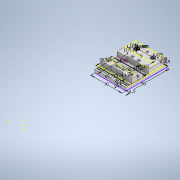
# Autodesk Inventor part: YAchseBasisteil
Saved by Autodesk Inventor 2021 (Build 250183000, 183)
## iProperties
Created: 2021-02-21
Part Number: YAchseBasisteil
Material: Generisch
Document SubType Name: Modeling
Designer: Kathrin H. Ulmer
Density: 1 g/cm^3
Appearance: Vorgabe
Author: Kathrin H. Ulmer
Autodesk Inventor part; units mm, degrees
ref_plane "YZ Plane" through (0, 0, 0) normal (1, 0, 0) x (0, 1, 0)
ref_plane "XZ Plane" through (0, 0, 0) normal (0, 1, 0) x (-1, 0, 0)
ref_plane "XY Plane" through (0, 0, 0) normal (0, 0, 1) x (1, 0, 0)
sketch "Skizze1" plane through (0, 0, 0) normal (0, 1, 0) x (-1, 0, 0)
  line L0 (28.961, -192.7131) -> (-41.039, -192.7131)
  line L1 (-41.039, -192.7131) -> (-41.039, -282.7131)
  line L2 (-41.039, -282.7131) -> (28.961, -282.7131)
  line L3 (28.961, -282.7131) -> (28.961, -192.7131)
  line L4 (28.961, -196.2131) -> (-41.039, -196.2131)
  line L5 (28.961, -204.2131) -> (-41.039, -204.2131)
  line L6 (28.961, -200.2131) -> (-41.039, -200.2131)
  line L7 (28.961, -246.7131) -> (-41.039, -246.7131)
  line L8 (28.961, -238.7131) -> (-41.039, -238.7131)
  line L9 (28.961, -242.7131) -> (-41.039, -242.7131)
  line L10 (28.961, -192.7131) -> (-41.039, -192.7131)
  line L11 (-41.039, -192.7131) -> (-41.039, -191.2131)
  line L12 (-41.039, -191.2131) -> (28.961, -191.2131)
  line L13 (28.961, -191.2131) -> (28.961, -192.7131)
  point P0 (0, 0)
  dimension "d0" = 70
  dimension "d1" = 90
  dimension "d206" = 3.5
  dimension "d207" = 8
  dimension "d220" = 4
  dimension "d221" = 54
  dimension "d222" = 8
  dimension "d223" = 4
  dimension "d255" = 36
  dimension "d282" = 70
  dimension "d283" = 1.5
  constraints: 28 end point, 12 point on line, 7 perpendicular, 4 parallel, 3 horizontal
  measures "d0" distance of L2.end L1.end
  measures "d1" distance of L1.end L0.end
  measures "d206" distance between parallel lines of L4 L0
  measures "d207" distance between parallel lines of L5 L4
  measures "d220" distance between parallel lines of L5 L6
  measures "d221" distance between parallel lines of L0 L7
  measures "d222" distance between parallel lines of L7 L8
  measures "d223" distance between parallel lines of L7 L9
  measures "d255" distance between parallel lines of L2 L7
  measures "d282" distance of L11.end L12.end
  measures "d283" distance of L10.end L11.end
extrude "Extrusion1" add sketch "Skizze1" along normal blind 7 contours L3 L4 L1 L0 | L3 L6 L1 L4 | L3 L5 L1 L6 | L3 L8 L1 L5 | L3 L9 L1 L8 | L3 L7 L1 L9 | L3 L2 L1 L7
sketch "Skizze2" plane through (0, 7, 0) normal (0, 1, 0) x (1, 0, 0)
  line L0 (41.039, 282.7131) -> (-28.961, 282.7131) projected
  line L1 (-28.961, 282.7131) -> (41.039, 282.7131)
  line L2 (41.039, 282.7131) -> (41.039, 258.7131)
  line L3 (41.039, 258.7131) -> (-28.961, 258.7131)
  line L4 (-28.961, 258.7131) -> (-28.961, 282.7131)
  circle A0 centre (-13.961, 268.7131) radius 4.5
  circle A1 centre (26.039, 268.7131) radius 4.5
  point P0 (0, 0)
  point P1 (41.039, 282.7131)
  dimension "d4" = 24
  dimension "d5" = 70
  dimension "d17" = 9
  dimension "d18" = 9
  dimension "d19" = 15
  dimension "d21" = 10
  dimension "d22" = 15
  dimension "d23" = 40
  dimension "d64" = 10
  constraints: 8 end point, 2 centre point, 2 parallel, 1 horizontal, 1 perpendicular
  measures "d4" distance of L1.end L2.end
  measures "d5" distance of L2.end L3.end
  measures "d17" diameter of A0
  measures "d18" diameter of A1
  measures "d19" distance from line of L4 A0.centre
  measures "d21" distance from line of L3 A1.centre
  measures "d22" distance from line of L2 A1.centre
  measures "d23" distance of A1.centre A0.centre
  measures "d64" distance from line of L3 A0.centre
extrude "Extrusion2" add sketch "Skizze2" along normal blind 10 contours L2 L3 L4 L0 | A0 | A1
sketch "Skizze4" plane through (0, 17, 0) normal (0, 1, 0) x (1, 0, 0)
  point P0 (0, 0)
sketch "Skizze5" plane through (-28.961, 7, -258.7131) normal (0, 0, 1) x (1, 0, 0)
  point P0 (28.961, -7)
sketch "Skizze6" plane through (0, 17, 0) normal (0, 1, 0) x (1, 0, 0)
  circle A0 centre (-11.961, 268.7131) radius 4.5
  line L0 (41.039, 282.7131) -> (-28.961, 282.7131) projected
  line L1 (-28.961, 282.7131) -> (-28.961, 258.7131) projected
  line L2 (-28.961, 258.7131) -> (41.039, 258.7131) projected
  point P0 (0, 0)
  dimension "d34" = 9
  dimension "d36" = 17
  dimension "d65" = 10
  constraints: 1 centre point
  measures "d34" diameter of A0
  measures "d36" distance from line of L1 A0.centre
  measures "d65" distance from line of L2 A0.centre
sketch "Skizze9" plane through (0, 17, 0) normal (0, 1, 0) x (1, 0, 0)
  point P0 (0, 0)
sketch "Skizze10" plane through (0, 17, 0) normal (0, 1, 0) x (1, 0, 0)
  circle A0 centre (24.039, 268.7131) radius 4.5
  line L0 (41.039, 258.7131) -> (41.039, 282.7131) projected
  line L1 (41.039, 282.7131) -> (-28.961, 282.7131) projected
  line L2 (-28.961, 282.7131) -> (-28.961, 258.7131) projected
  point P0 (0, 0)
  dimension "d37" = 9
  dimension "d38" = 17
  dimension "d39" = 14
  dimension "d40" = 70
  constraints: 1 centre point
  measures "d37" diameter of A0
  measures "d38" distance from line of L0 A0.centre
  measures "d39" distance from line of L1 A0.centre
  measures "d40" distance between parallel lines of L0 L2
sketch "Skizze11" plane through (0, 17, 0) normal (0, 1, 0) x (1, 0, 0)
  point P0 (0, 0)
extrude "Extrusion6" cut sketch "Skizze6" against normal blind 14
sketch "Skizze16" plane through (0, 17, 0) normal (0, 1, 0) x (1, 0, 0)
  line L0 (41.039, 282.7131) -> (-28.961, 282.7131) projected
  line L1 (-28.961, 258.7131) -> (41.039, 258.7131) projected
  point P0 (0, 0)
  dimension "d63" = 24
  measures "d63" distance between parallel lines of L0 L1
extrude "Extrusion11" cut sketch "Skizze10" against normal blind 13.75
sketch "Skizze17" plane through (41.039, 0, -192.7131) normal (1, 0, 0) x (0, 0, -1)
  line L0 (86.5, 13) -> (84, 13)
  line L1 (84, 13) -> (84, 7.5)
  line L2 (84, 7.5) -> (86.5, 7.5)
  line L3 (86.5, 7.5) -> (86.5, 13)
  line L4 (90, 0) -> (90, 17) projected
  line L5 (66, 17) -> (90, 17) projected
  point P0 (-192.7131, 0)
  dimension "d68" = 2.5
  dimension "d69" = 5.5
  dimension "d70" = 3.5
  dimension "d71" = 4
  constraints: 8 end point, 2 parallel, 1 horizontal, 1 perpendicular
  measures "d68" distance of L2.end L1.end
  measures "d69" distance of L1.end L0.end
  measures "d70" distance between parallel lines of L4 L3
  measures "d71" distance between parallel lines of L5 L0
extrude "Extrusion12" cut sketch "Skizze17" against normal blind 23
sketch "Skizze18" plane through (-28.961, 0, -282.7131) normal (-1, 0, 0) x (0, 0, 1)
  line L0 (3.5, 7.5) -> (6, 7.5)
  line L1 (6, 7.5) -> (6, 13)
  line L2 (6, 13) -> (3.5, 13)
  line L3 (3.5, 13) -> (3.5, 7.5)
  line L4 (0, 17) -> (24, 17) projected
  line L5 (0, 0) -> (0, 17) projected
  point P0 (282.7131, 0)
  dimension "d74" = 2.5
  dimension "d75" = 5.5
  dimension "d76" = 4
  dimension "d77" = 3.5
  constraints: 8 end point, 2 parallel, 1 horizontal, 1 perpendicular
  measures "d74" distance of L2.end L1.end
  measures "d75" distance of L1.end L0.end
  measures "d76" distance between parallel lines of L4 L2
  measures "d77" distance between parallel lines of L5 L3
extrude "Extrusion13" cut sketch "Skizze18" against normal blind 23
sketch "Skizze19" plane through (41.039, 0, -282.7131) normal (0, 0, -1) x (-1, 0, 0)
  circle A0 centre (53, 10.125) radius 2.125
  line L0 (70, 0) -> (70, 17) projected
  line L1 (0, 17) -> (70, 17) projected
  circle A1 centre (17, 10.125) radius 2.125
  line L2 (0, 0) -> (0, 17) projected
  point P0 (41.039, 0)
  dimension "d80" = 4.25
  dimension "d81" = 17
  dimension "d82" = 6.875
  dimension "d83" = 4.25
  dimension "d84" = 6.875
  dimension "d85" = 17
  constraints: 2 centre point
  measures "d80" diameter of A0
  measures "d81" distance from line of L0 A0.centre
  measures "d82" distance from line of L1 A0.centre
  measures "d83" diameter of A1
  measures "d84" distance from line of L1 A1.centre
  measures "d85" distance from line of L2 A1.centre
extrude "Extrusion14" cut sketch "Skizze19" against normal blind 30 contours A1
extrude "Extrusion15" cut sketch "Skizze19" against normal blind 30 contours A0
sketch "Skizze20" plane through (41.039, 0, -282.7131) normal (0, 0, -1) x (-1, 0, 0)
  circle A0 centre (8, 10.125) radius 2.25
  line L0 (0, 17) -> (70, 17) projected
  line L1 (0, 0) -> (0, 17) projected
  circle A1 centre (62, 10.125) radius 2.125
  line L2 (70, 0) -> (70, 17) projected
  point P0 (41.039, 0)
  dimension "d90" = 4.5
  dimension "d91" = 6.875
  dimension "d92" = 8
  dimension "d93" = 4.25
  dimension "d94" = 6.875
  dimension "d95" = 8
  constraints: 2 centre point
  measures "d90" diameter of A0
  measures "d91" distance from line of L0 A0.centre
  measures "d92" distance from line of L1 A0.centre
  measures "d93" diameter of A1
  measures "d94" distance from line of L0 A1.centre
  measures "d95" distance from line of L2 A1.centre
extrude "Extrusion16" cut sketch "Skizze20" against normal blind 30 contours A0
extrude "Extrusion17" cut sketch "Skizze20" against normal blind 30 contours A1
sketch "Skizze21" plane through (0, 7, 0) normal (0, 1, 0) x (1, 0, 0)
  line L0 (-28.961, 282.7131) -> (-28.961, 192.7131) projected
  line L1 (41.039, 192.7131) -> (41.039, 282.7131) projected
  line L2 (-86.883, 193.3511) -> (41.039, 193.3511)
  line L3 (41.039, 193.3511) -> (41.039, 216.8511)
  line L4 (41.039, 216.8511) -> (-86.883, 216.8511)
  line L5 (-86.883, 216.8511) -> (-86.883, 193.3511)
  line L6 (-86.883, 216.8511) -> (-16.883, 216.8511)
  line L7 (-16.883, 216.8511) -> (-16.883, 208.3511)
  line L8 (41.039, 206.8012) -> (-28.961, 206.8012)
  line L9 (-86.883, 208.3511) -> (-86.883, 216.8511)
  line L10 (-28.961, 206.8012) -> (-6.961, 206.8012)
  line L11 (-6.961, 206.8012) -> (-6.961, 204.8012)
  line L12 (-6.961, 204.8012) -> (-28.961, 204.8012)
  line L13 (-28.961, 204.8012) -> (-28.961, 206.8012)
  line L14 (41.039, 206.8012) -> (19.039, 206.8012)
  line L15 (19.039, 206.8012) -> (19.039, 204.8012)
  line L16 (19.039, 204.8012) -> (41.039, 204.8012)
  line L17 (41.039, 204.8012) -> (41.039, 206.8012)
  line L18 (-86.883, 204.8511) -> (41.039, 204.8511)
  line L19 (-86.883, 196.8511) -> (41.039, 196.8511)
  point P0 (0, 0)
  point P1 (41.039, 206.8012)
  point P2 (-28.961, 216.8511)
  point P3 (-28.961, 206.8012)
  point P4 (-28.961, 204.8012)
  point P5 (41.039, 204.8012)
  point P6 (41.039, 216.8511)
  dimension "d101" = 8.5
  dimension "d102" = 22
  dimension "d103" = 2
  dimension "d104" = 22
  dimension "d105" = 2
  dimension "d203" = 0.0499
  dimension "d204" = 8
  dimension "d205" = 3.5
  dimension "d286" = 13.4501
  constraints: 36 end point, 8 parallel, 6 perpendicular, 4 horizontal, 4 point on line
  measures "d101" distance of L7.end L6.end
  measures "d102" distance of L11.end L12.end
  measures "d103" distance between parallel lines of L12 L8
  measures "d104" distance of L16.end L15.end
  measures "d105" distance of L15.end L14.end
  measures "d203" distance between parallel lines of L12 L18
  measures "d204" distance between parallel lines of L18 L19
  measures "d205" distance between parallel lines of L2 L19
  measures "d286" distance between parallel lines of L2 L8
sketch "Skizze22" plane through (0, 7, 0) normal (0, 1, 0) x (1, 0, 0)
  line L0 (-22.961, 228.2131) -> (-17.861, 228.2131)
  line L1 (-17.861, 228.2131) -> (-17.861, 222.7131)
  line L2 (-17.861, 222.7131) -> (-22.961, 222.7131)
  line L3 (-22.961, 222.7131) -> (-22.961, 228.2131)
  line L4 (-3.861, 228.2131) -> (1.239, 228.2131)
  line L5 (1.239, 228.2131) -> (1.239, 222.7131)
  line L6 (1.239, 222.7131) -> (-3.861, 222.7131)
  line L7 (-3.861, 222.7131) -> (-3.861, 228.2131)
  line L8 (10.839, 228.2131) -> (15.939, 228.2131)
  line L9 (15.939, 228.2131) -> (15.939, 222.7131)
  line L10 (15.939, 222.7131) -> (10.839, 222.7131)
  line L11 (10.839, 222.7131) -> (10.839, 228.2131)
  line L12 (29.939, 228.2131) -> (35.039, 228.2131)
  line L13 (35.039, 228.2131) -> (35.039, 222.7131)
  line L14 (35.039, 222.7131) -> (29.939, 222.7131)
  line L15 (29.939, 222.7131) -> (29.939, 228.2131)
  line L16 (-28.961, 258.7131) -> (-28.961, 192.7131) projected
  line L17 (41.039, 192.7131) -> (41.039, 258.7131) projected
  line L18 (-28.961, 192.7131) -> (41.039, 192.7131) projected
  point P0 (0, 0)
  dimension "d120" = 5.1
  dimension "d121" = 5.5
  dimension "d122" = 5.1
  dimension "d123" = 5.1
  dimension "d124" = 5.1
  dimension "d125" = 6
  dimension "d126" = 6
  dimension "d127" = 14
  dimension "d128" = 14
  dimension "d161" = 30
  constraints: 32 end point, 8 parallel, 6 point on line, 4 horizontal, 4 perpendicular
  measures "d120" distance of L1.end L2.end
  measures "d121" distance of L0.end L1.end
  measures "d122" distance of L5.end L6.end
  measures "d123" distance of L9.end L10.end
  measures "d124" distance of L13.end L14.end
  measures "d125" distance between parallel lines of L16 L3
  measures "d126" distance between parallel lines of L17 L13
  measures "d127" distance between parallel lines of L15 L9
  measures "d128" distance between parallel lines of L1 L7
  measures "d161" distance between parallel lines of L18 L2
extrude "Extrusion22" add sketch "Skizze21" along normal blind 10 contours L4 L1 L8 L0
extrude "Extrusion23" add sketch "Skizze21" along normal blind 10 contours L8 L11 L18 L0 | L18 L11 L12 L0 | L8 L1 L18 L15 | L18 L1 L16 L15
sketch "Skizze25" plane through (0, 17, 0) normal (0, 1, 0) x (1, 0, 0)
  line L0 (-22.961, 214.8511) -> (-17.861, 214.8511)
  line L1 (-17.861, 214.8511) -> (-17.861, 210.6011)
  line L2 (-17.861, 210.6011) -> (-22.961, 210.6011)
  line L3 (-22.961, 210.6011) -> (-22.961, 214.8511)
  line L4 (-3.861, 214.8511) -> (1.239, 214.8511)
  line L5 (1.239, 214.8511) -> (1.239, 210.6011)
  line L6 (1.239, 210.6011) -> (-3.861, 210.6011)
  line L7 (-3.861, 210.6011) -> (-3.861, 214.8511)
  line L8 (10.839, 214.8511) -> (15.939, 214.8511)
  line L9 (15.939, 214.8511) -> (15.939, 210.6011)
  line L10 (15.939, 210.6011) -> (10.839, 210.6011)
  line L11 (10.839, 210.6011) -> (10.839, 214.8511)
  line L12 (29.939, 214.8511) -> (35.039, 214.8511)
  line L13 (35.039, 214.8511) -> (35.039, 210.6011)
  line L14 (35.039, 210.6011) -> (29.939, 210.6011)
  line L15 (29.939, 210.6011) -> (29.939, 214.8511)
  line L16 (-28.961, 216.8511) -> (-28.961, 204.8012) projected
  line L17 (41.039, 204.8012) -> (41.039, 216.8511) projected
  line L18 (41.039, 216.8511) -> (-28.961, 216.8511) projected
  point P0 (0, 0)
  point P1 (41.039, 216.2131)
  dimension "d141" = 5.1
  dimension "d142" = 4.25
  dimension "d143" = 5.1
  dimension "d144" = 4.25
  dimension "d145" = 5.1
  dimension "d146" = 4.25
  dimension "d147" = 5.1
  dimension "d148" = 4.25
  dimension "d149" = 6
  dimension "d150" = 14
  dimension "d151" = 6
  dimension "d152" = 14
  dimension "d153" = 2
  dimension "d154" = 2
  dimension "d155" = 2
  constraints: 32 end point, 8 parallel, 4 horizontal, 4 perpendicular, 1 point on line, 1 other
  measures "d141" distance of L1.end L2.end
  measures "d142" distance of L0.end L1.end
  measures "d143" distance of L5.end L6.end
  measures "d144" distance of L4.end L5.end
  measures "d145" distance of L9.end L10.end
  measures "d146" distance of L8.end L9.end
  measures "d147" distance of L13.end L14.end
  measures "d148" distance of L12.end L13.end
  measures "d149" distance between parallel lines of L16 L3
  measures "d150" distance between parallel lines of L7 L1
  measures "d151" distance between parallel lines of L17 L13
  measures "d152" distance between parallel lines of L9 L15
extrude "Extrusion24" cut sketch "Skizze25" against normal blind 30
sketch "Skizze27" plane through (0, 7, 0) normal (0, 1, 0) x (1, 0, 0)
  point P0 (0, 0)
sketch "Skizze28" plane through (0, 7, 0) normal (0, 1, 0) x (1, 0, 0)
  line L0 (-28.961, 258.7131) -> (-28.961, 216.8511) projected
  line L1 (41.039, 216.8511) -> (41.039, 258.7131) projected
  line L2 (-28.961, 253.3551) -> (41.039, 253.3551)
  line L3 (41.039, 253.3551) -> (41.039, 229.6051)
  line L4 (41.039, 229.6051) -> (-28.961, 229.6051)
  line L5 (-28.961, 229.6051) -> (-28.961, 253.3551)
  line L6 (41.039, 216.8511) -> (-28.961, 216.8511) projected
  line L7 (-28.961, 192.7131) -> (41.039, 192.7131) projected
  line L8 (-28.961, 204.8012) -> (-6.961, 204.8012) projected
  line L9 (-6.961, 206.8012) -> (19.039, 206.8012) projected
  line L10 (19.039, 204.8012) -> (41.039, 204.8012) projected
  line L11 (-28.961, 253.3551) -> (41.039, 253.3551)
  line L12 (41.039, 253.3551) -> (41.039, 244.8551)
  line L13 (41.039, 244.8551) -> (-28.961, 244.8551)
  line L14 (-28.961, 244.8551) -> (-28.961, 253.3551)
  line L15 (41.039, 204.8012) -> (41.039, 216.8511) projected
  line L16 (41.039, 244.8551) -> (19.039, 244.8551)
  line L17 (19.039, 244.8551) -> (19.039, 242.8551)
  line L18 (19.039, 242.8551) -> (41.039, 242.8551)
  line L19 (41.039, 242.8551) -> (41.039, 244.8551)
  line L20 (-28.961, 244.8551) -> (-6.961, 244.8551)
  line L21 (-6.961, 244.8551) -> (-6.961, 242.8551)
  line L22 (-6.961, 242.8551) -> (-28.961, 242.8551)
  line L23 (-28.961, 242.8551) -> (-28.961, 244.8551)
  point P0 (0, 0)
  point P1 (41.039, 253.3551)
  point P2 (-28.961, 242.8551)
  point P3 (41.039, 242.8551)
  point P4 (-28.961, 253.3551)
  dimension "d162" = 23.75
  dimension "d163" = 12.754
  dimension "d164" = 12.0881
  dimension "d165" = 14.0881
  dimension "d166" = 12.0499
  dimension "d167" = 8.5
  dimension "d168" = 10.0499
  dimension "d169" = 22
  dimension "d170" = 22
  dimension "d171" = 2
  dimension "d172" = 22
  dimension "d173" = 2
  dimension "d202" = 15.25
  constraints: 32 end point, 8 parallel, 4 horizontal, 4 perpendicular, 1 point on line
  measures "d162" distance between parallel lines of L4 L2
  measures "d163" distance between parallel lines of L4 L6
  measures "d164" distance between parallel lines of L7 L8
  measures "d165" distance between parallel lines of L7 L9
  measures "d166" distance between parallel lines of L10 L6
  measures "d167" distance between parallel lines of L13 L2
  measures "d168" distance between parallel lines of L9 L6
  measures "d169" distance from line of L10.start L15
  measures "d170" distance of L18.end L17.end
  measures "d171" distance of L17.end L16.end
  measures "d172" distance of L21.end L22.end
  measures "d173" distance of L20.end L21.end
  measures "d202" distance between parallel lines of L4 L13
sketch "Skizze30" plane through (0, 7, 0) normal (0, 1, 0) x (1, 0, 0)
  point P0 (0, 0)
extrude "Extrusion26" add sketch "Skizze28" along normal blind 10 contours L2 L1 L13 L0 | L13 L21 L22 L0 | L1 L18 L17 L13
sketch "Skizze31" plane through (0, 17, 0) normal (0, 1, 0) x (1, 0, 0)
  line L0 (-3.861, 33.1581) -> (1.239, 33.1581)
  line L1 (1.239, 33.1581) -> (1.239, 28.9081)
  line L2 (1.239, 28.9081) -> (-3.861, 28.9081)
  line L3 (-3.861, 28.9081) -> (-3.861, 33.1581)
  line L4 (10.839, 33.1581) -> (15.939, 33.1581)
  line L5 (15.939, 33.1581) -> (15.939, 28.9081)
  line L6 (15.939, 28.9081) -> (10.839, 28.9081)
  line L7 (10.839, 28.9081) -> (10.839, 33.1581)
  line L8 (41.039, 242.8551) -> (41.039, 253.3551) projected
  line L9 (-28.961, 253.3551) -> (-28.961, 242.8551) projected
  line L10 (-6.961, 204.8012) -> (-6.961, 206.8012) projected
  line L11 (19.039, 206.8012) -> (19.039, 204.8012) projected
  line L12 (19.039, 244.8551) -> (19.039, 242.8551) projected
  line L13 (-6.961, 242.8551) -> (-6.961, 244.8551) projected
  point P0 (0, 0)
  point P1 (-28.961, 250.7131)
  dimension "d190" = 5.1
  dimension "d191" = 4.25
  dimension "d192" = 5.1
  dimension "d193" = 4.25
  dimension "d194" = 25.1
  dimension "d195" = 25.1
  dimension "d196" = 26
  dimension "d197" = 26
  constraints: 16 end point, 4 parallel, 2 horizontal, 2 perpendicular
  measures "d190" distance of L1.end L2.end
  measures "d191" distance of L0.end L1.end
  measures "d192" distance of L5.end L6.end
  measures "d193" distance of L4.end L5.end
  measures "d194" distance between parallel lines of L8 L5
  measures "d195" distance between parallel lines of L9 L3
  measures "d196" distance between parallel lines of L10 L11
  measures "d197" distance between parallel lines of L12 L13
extrude "Extrusion28" cut sketch "Skizze31" against normal blind 30
extrude "Extrusion29" cut sketch "Skizze22" against normal blind 30
sketch "Skizze32" plane through (0, 17, 0) normal (0, 1, 0) x (1, 0, 0)
  line L0 (-3.861, 248.054) -> (1.239, 248.054)
  line L1 (1.239, 248.054) -> (1.239, 252.054)
  line L2 (1.239, 252.054) -> (-3.861, 252.054)
  line L3 (-3.861, 252.054) -> (-3.861, 248.054)
  line L4 (10.839, 248.054) -> (15.939, 248.054)
  line L5 (15.939, 248.054) -> (15.939, 252.054)
  line L6 (15.939, 252.054) -> (10.839, 252.054)
  line L7 (10.839, 252.054) -> (10.839, 248.054)
  line L8 (-28.961, 282.7131) -> (-28.961, 258.7131) projected
  line L9 (41.039, 258.7131) -> (41.039, 282.7131) projected
  line L10 (-6.961, 244.8551) -> (19.039, 244.8551) projected
  line L11 (-28.961, 242.4631) -> (41.039, 242.4631)
  line L12 (-28.961, 258.7131) -> (-28.961, 216.8511) projected
  line L13 (-6.961, 244.4631) -> (-6.961, 242.4631)
  line L14 (19.039, 244.4631) -> (19.039, 242.4631)
  line L15 (-10.545, 205.4869) -> (-10.545, 192.7131)
  line L16 (-28.961, 192.7131) -> (41.039, 192.7131) projected
  line L17 (-28.961, 199.3012) -> (41.039, 199.3012)
  line L18 (19.039, 204.8012) -> (41.039, 204.8012) projected
  line L19 (-28.961, 236.9631) -> (41.039, 236.9631)
  line L20 (-28.961, 258.7131) -> (41.039, 258.7131) projected
  line L21 (-6.961, 244.4631) -> (19.039, 244.4631)
  line L22 (-28.961, 258.7131) -> (41.039, 258.7131)
  line L23 (41.039, 258.7131) -> (41.039, 242.4631)
  line L24 (41.039, 242.4631) -> (-28.961, 242.4631)
  line L25 (-28.961, 242.4631) -> (-28.961, 258.7131)
  line L26 (-6.961, 244.4631) -> (19.039, 244.4631)
  line L27 (19.039, 244.4631) -> (19.039, 242.4631)
  line L28 (19.039, 242.4631) -> (-6.961, 242.4631)
  line L29 (-6.961, 242.4631) -> (-6.961, 244.4631)
  point P0 (0, 0)
  point P1 (-28.961, 242.8551)
  point P2 (41.039, 242.8551)
  dimension "d208" = 5.1
  dimension "d209" = 4
  dimension "d210" = 5.1
  dimension "d211" = 4
  dimension "d212" = 25.1
  dimension "d213" = 25.1
  dimension "d214" = 3.1988
  dimension "d215" = 3.1988
  dimension "d256" = 12.7738
  dimension "d257" = 5.5
  dimension "d258" = 5.5
  dimension "d259" = 37.6619
  dimension "d260" = 16.25
  dimension "d261" = 2
  constraints: 46 end point, 10 parallel, 7 horizontal, 4 perpendicular, 4 point on line
  measures "d208" distance of L2.end L1.end
  measures "d209" distance of L1.end L0.end
  measures "d210" distance of L6.end L5.end
  measures "d211" distance of L5.end L4.end
  measures "d212" distance between parallel lines of L8 L3
  measures "d213" distance between parallel lines of L9 L5
  measures "d214" distance between parallel lines of L10 L4
  measures "d215" distance from line of L0.end L10
  measures "d256" distance of L15.start L15.end
  measures "d257" distance between parallel lines of L18 L17
  measures "d258" distance between parallel lines of L19 L11
  measures "d259" distance between parallel lines of L17 L19
  measures "d260" distance between parallel lines of L20 L11
  measures "d261" distance between parallel lines of L11 L21
extrude "Extrusion30" cut sketch "Skizze32" against normal blind 30 contours L3 L2 L1 L0 | L7 L6 L5 L4
sketch "Skizze33" plane through (0, 17, 0) normal (0, 1, 0) x (1, 0, 0)
  line L0 (41.039, 216.8511) -> (-28.961, 216.8511) projected
  line L1 (-28.961, 192.7131) -> (41.039, 192.7131) projected
  line L2 (19.039, 242.8551) -> (41.039, 242.8551) projected
  point P0 (0, 0)
  point P1 (41.039, 216.2131)
  point P2 (-28.961, 216.8511)
  dimension "d218" = 24.138
  dimension "d219" = 50.142
  constraints: 1 other
  measures "d219" distance between parallel lines of L2 L1
sketch "Skizze34" plane through (0, 17, 0) normal (0, 1, 0) x (1, 0, 0)
  point P0 (0, 0)
sketch "Skizze35" plane through (41.039, 0, -282.7131) normal (0, 0, -1) x (-1, 0, 0)
  circle A0 centre (62, 10.125) radius 2.125 projected
  line L0 (62, 10.125) -> (62, 17)
  line L1 (0, 17) -> (70, 17) projected
  line L2 (53.0937, 10.125) -> (53.0937, 17)
  line L3 (17.1042, 10.125) -> (17.1042, 17)
  line L4 (62, 10.125) -> (70, 10.125)
  line L5 (53.0937, 10.125) -> (70, 10.125)
  line L6 (8.0195, 10.125) -> (0, 10.125)
  point P0 (41.039, 0)
  dimension "d141" = 5.1
  dimension "d142" = 4.25
  dimension "d143" = 5.1
  dimension "d144" = 4.25
  dimension "d145" = 5.1
  dimension "d146" = 4.25
  dimension "d147" = 5.1
  dimension "d148" = 4.25
  dimension "d149" = 6
  dimension "d150" = 14
  dimension "d151" = 6
  dimension "d152" = 14
  dimension "d153" = 2
  dimension "d154" = 2
  dimension "d155" = 2
  dimension "d224" = 8
  dimension "d225" = 16.9063
  dimension "d226" = 8.0195
  dimension "d227" = 17.1042
  dimension "d229" = 6.875
  dimension "d230" = 6.875
  constraints: 12 end point, 3 point on line, 2 horizontal, 2 parallel, 1 vertical
  measures "d224" distance of L0.start L4.end
  measures "d225" distance of L2.start L4.end
  measures "d226" distance of L6.start L6.end
  measures "d227" distance of L6.end L3.start
  measures "d229" distance of L3.start L3.end
  measures "d230" distance of L2.start L2.end
sketch "Skizze36" plane through (-28.961, 0, -282.7131) normal (-1, 0, 0) x (0, 0, 1)
  line L0 (0, 17) -> (24, 17) projected
  line L1 (0, 0) -> (90, 0) projected
  point P0 (282.7131, 0)
  point P1 (39.858, 17)
  dimension "d228" = 17
  measures "d228" distance between parallel lines of L0 L1
sketch "Skizze37" plane through (41.039, 0, -282.7131) normal (0, 0, -1) x (-1, 0, 0)
  circle A0 centre (35, 8.5) radius 4.5
  line L0 (0, 17) -> (70, 17) projected
  circle A1 centre (17, 10.125) radius 2.125 projected
  point P0 (41.039, 0)
  dimension "d231" = 9
  dimension "d232" = 8.5
  dimension "d233" = 18
  constraints: 1 centre point
  measures "d231" diameter of A0
  measures "d232" distance from line of L0 A0.centre
  measures "d233" horizontal distance of A1.centre A0.centre
extrude "Extrusion31" cut sketch "Skizze37" against normal blind 20 contours A0
sketch "Skizze38" plane through (41.039, 0, -282.7131) normal (0, 0, -1) x (-1, 0, 0)
  line L0 (37.5, 16) -> (32, 16)
  line L1 (32, 16) -> (32, 13.5)
  line L2 (32, 13.5) -> (37.5, 13.5)
  line L3 (37.5, 13.5) -> (37.5, 16)
  line L4 (0, 17) -> (70, 17) projected
  circle A0 centre (17, 10.125) radius 2.125 projected
  point P0 (41.039, 0)
  dimension "d236" = 5.5
  dimension "d237" = 2.5
  dimension "d238" = 1
  dimension "d239" = 15
  constraints: 8 end point, 2 parallel, 1 horizontal, 1 perpendicular
  measures "d236" distance of L2.end L1.end
  measures "d237" distance of L1.end L0.end
  measures "d238" distance between parallel lines of L4 L0
  measures "d239" distance from line of A0.centre L1
sketch "Skizze39" plane through (0, 17, 0) normal (0, 1, 0) x (1, 0, 0)
  line L0 (41.039, 282.7131) -> (-28.961, 282.7131) projected
  line L1 (3.6174, 282.7131) -> (3.6174, 259.2524)
  line L2 (9.1174, 282.7131) -> (9.1174, 259.2524)
  line L3 (9.1174, 259.2524) -> (9.1174, 259.2524)
  line L4 (3.6174, 274.7131) -> (9.1174, 274.7131)
  circle A0 centre (6.3674, 274.7131) radius 2.05
  point P0 (0, 0)
  dimension "d240" = 5.5
  dimension "d241" = 4.1
  dimension "d242" = 8
  constraints: 8 end point, 4 point on line, 1 centre point, 1 horizontal, 1 midpoint, 1 perpendicular, 1 vertical
  measures "d240" distance between parallel lines of L2 L1
  measures "d241" diameter of A0
  measures "d242" distance from line of L0 A0.centre
extrude "Extrusion32" cut sketch "Skizze39" against normal blind 6 contours A0 L4 | L4 A0
extrude "Extrusion33" cut sketch "Skizze38" against normal blind 12 contours L3 L2 L1 L0
sketch "Skizze40" plane through (41.039, 17, -216.8511) normal (0, 0, -1) x (-1, 0, 0)
  point P0 (41.039, -17)
sketch "Skizze41" plane through (-6.961, 7, -206.8012) normal (0, 0, 1) x (1, 0, 0)
  line L0 (8.2, 10) -> (8.2, -7) projected
  circle A0 centre (12.6732, 5.2496) radius 2
  point P0 (6.961, -7)
  point P1 (8.2, 0)
  dimension "d247" = 4
  constraints: 1 centre point
  measures "d247" diameter of A0
extrude "Extrusion34" cut sketch "Skizze41" against normal blind 15
sketch "Skizze42" plane through (0, 17, 0) normal (0, 1, 0) x (1, 0, 0)
  line L0 (3.7122, 206.8012) -> (3.7122, 216.8511) projected
  line L1 (2.979, 211.3804) -> (8.479, 211.3804)
  line L2 (8.479, 211.3804) -> (8.479, 213.8804)
  line L3 (8.479, 213.8804) -> (2.979, 213.8804)
  line L4 (2.979, 213.8804) -> (2.979, 211.3804)
  line L5 (2.979, 212.6304) -> (8.479, 212.6304)
  line L6 (5.729, 211.3804) -> (5.729, 213.8804)
  line L7 (10.839, 210.6011) -> (10.839, 214.8511) projected
  line L8 (7.7302, 211.8307) -> (7.7122, 221.902)
  line L9 (7.7122, 206.8012) -> (7.7122, 216.8511) projected
  line L10 (3.7122, 214.0015) -> (7.7122, 214.0087)
  line L11 (5.7122, 214.0051) -> (5.7122, 227.9631)
  line L12 (41.039, 216.8511) -> (-28.961, 216.8511) projected
  point P0 (0, 0)
  point P1 (41.039, 216.2131)
  point P2 (-28.961, 216.8511)
  dimension "d250" = 5.5
  dimension "d251" = 2.5
  dimension "d252" = 2.36
  constraints: 18 end point, 4 midpoint, 2 parallel, 2 perpendicular, 1 horizontal, 1 point on line, 1 vertical, 1 other
  measures "d250" distance of L3.end L2.end
  measures "d251" distance of L2.end L1.end
  measures "d252" distance between parallel lines of L7 L2
extrude "Extrusion35" cut sketch "Skizze42" against normal blind 20 contours L3 L6 L5 L0 | L0 L5 L4 L3 | L5 L6 L1 L0 | L0 L1 L4 L5 | L3 L9 L5 L6 | L5 L9 L1 L6 | L3 L8 L5 L9 | L5 L2 L1 L9 | L3 L2 L5 L8
sketch "Skizze43" plane through (0, 7, 0) normal (0, 1, 0) x (1, 0, 0)
  point P0 (0, 0)
sketch "Skizze44" plane through (0, 7, 0) normal (0, 1, 0) x (1, 0, 0)
  line L0 (-28.961, 282.7131) -> (-28.961, 192.7131) projected
  line L1 (-28.961, 241.7252) -> (41.039, 241.7252)
  line L2 (41.039, 192.7131) -> (41.039, 282.7131) projected
  line L3 (-28.961, 199.3012) -> (41.039, 199.3012)
  line L4 (-28.961, 204.8012) -> (-6.961, 204.8012) projected
  line L5 (-28.961, 192.7131) -> (41.039, 192.7131) projected
  line L6 (-6.961, 243.7252) -> (19.039, 243.7252)
  line L7 (19.039, 243.7252) -> (19.039, 241.7252)
  line L8 (19.039, 241.7252) -> (-6.961, 241.7252)
  line L9 (-6.961, 241.7252) -> (-6.961, 243.7252)
  line L10 (-6.961, 244.8551) -> (19.039, 244.8551)
  line L11 (19.039, 244.8551) -> (19.039, 243.7252)
  line L12 (19.039, 243.7252) -> (-6.961, 243.7252)
  line L13 (-6.961, 243.7252) -> (-6.961, 244.8551)
  line L14 (-28.961, 242.8551) -> (-28.961, 216.8511) projected
  line L15 (-28.961, 242.8551) -> (-6.961, 242.8551)
  line L16 (-6.961, 242.8551) -> (-6.961, 241.7252)
  line L17 (-6.961, 241.7252) -> (-28.961, 241.7252)
  line L18 (-28.961, 241.7252) -> (-28.961, 242.8551)
  line L19 (41.039, 241.7252) -> (19.039, 241.7252)
  line L20 (19.039, 241.7252) -> (19.039, 242.8551)
  line L21 (19.039, 242.8551) -> (41.039, 242.8551)
  line L22 (41.039, 242.8551) -> (41.039, 241.7252)
  point P0 (0, 0)
  dimension "d262" = 5.5
  dimension "d263" = 6.5881
  dimension "d264" = 42.424
  dimension "d265" = 2
  constraints: 36 end point, 8 parallel, 5 horizontal, 4 perpendicular, 3 point on line
  measures "d262" distance between parallel lines of L4 L3
  measures "d263" distance between parallel lines of L5 L3
  measures "d264" distance between parallel lines of L3 L1
  measures "d265" distance between parallel lines of L1 L6
sketch "Skizze45" plane through (0, 7, 0) normal (0, 1, 0) x (1, 0, 0)
  line L0 (41.039, 258.7131) -> (-28.961, 258.7131) projected
  line L1 (41.039, 258.7131) -> (-28.961, 258.7131)
  line L2 (-28.961, 258.7131) -> (-28.961, 242.4631)
  line L3 (-28.961, 242.4631) -> (41.039, 242.4631)
  line L4 (41.039, 242.4631) -> (41.039, 258.7131)
  point P0 (0, 0)
  dimension "d266" = 70
  dimension "d267" = 16.25
  constraints: 8 end point, 2 parallel, 1 horizontal, 1 perpendicular
  measures "d266" distance of L3.end L2.end
  measures "d267" distance of L2.end L1.end
extrude "Extrusion36" add sketch "Skizze45" along normal blind 10
sketch "Skizze46" plane through (0, 17, 0) normal (0, 1, 0) x (1, 0, 0)
  line L0 (-6.961, 206.8012) -> (-6.961, 204.8012) projected
  line L1 (-6.961, 204.8012) -> (-6.961, 243.3573)
  line L2 (19.039, 204.8012) -> (19.039, 206.8012) projected
  line L3 (19.039, 204.8012) -> (19.039, 242.4454)
  line L4 (41.039, 242.4631) -> (-28.961, 242.4631) projected
  line L5 (-6.961, 242.4631) -> (19.039, 242.4631)
  line L6 (19.039, 242.4631) -> (19.039, 244.4631)
  line L7 (19.039, 244.4631) -> (-6.961, 244.4631)
  line L8 (-6.961, 244.4631) -> (-6.961, 242.4631)
  line L9 (-3.861, 252.054) -> (-3.861, 248.054) projected
  line L10 (-3.861, 248.054) -> (1.239, 248.054) projected
  line L11 (-3.8399, 250.2903) -> (1.2601, 250.2903)
  line L12 (1.2601, 250.2903) -> (1.2601, 246.3588)
  line L13 (1.2601, 246.3588) -> (-3.8399, 246.3588)
  line L14 (-3.8399, 246.3588) -> (-3.8399, 250.2903)
  line L15 (15.939, 252.054) -> (10.839, 252.054) projected
  line L16 (15.939, 248.054) -> (15.939, 252.054) projected
  line L17 (10.8601, 250.2903) -> (15.9601, 250.2903)
  line L18 (15.9601, 250.2903) -> (15.9601, 246.3588)
  line L19 (15.9601, 246.3588) -> (10.8601, 246.3588)
  line L20 (10.8601, 246.3588) -> (10.8601, 250.2903)
  point P0 (0, 0)
  point P1 (19.039, 242.4631)
  point P2 (19.039, 242.4631)
  point P3 (19.039, 243.3573)
  dimension "d270" = 26
  dimension "d271" = 2
  dimension "d272" = 5.3543
  constraints: 28 end point, 6 parallel, 3 horizontal, 3 perpendicular, 2 point on line, 2 vertical
  measures "d270" distance of L7.end L6.end
  measures "d271" distance of L6.end L5.end
  measures "d272" distance of L10.end L13.end
extrude "Extrusion37" cut sketch "Skizze46" against normal blind 50 contours L11 L12 L13 L14
extrude "Extrusion38" cut sketch "Skizze46" against normal blind 50 contours L17 L18 L19 L20
extrude "Extrusion39" cut sketch "Skizze46" against normal blind 10 contours L1 L8 L7 L6 L4
sketch "Skizze47" plane through (0, 7, 0) normal (0, 1, 0) x (1, 0, 0)
  line L0 (-28.6934, 236.0511) -> (41.039, 236.0511)
  line L1 (41.039, 192.7131) -> (41.039, 282.7131) projected
  line L2 (-28.961, 241.5511) -> (-6.961, 241.5511) projected
  line L3 (-28.961, 282.7131) -> (-28.961, 192.7131) projected
  line L4 (-28.961, 199.4749) -> (41.039, 199.4749)
  point P0 (0, 0)
  dimension "d279" = 5.5
  dimension "d280" = 69.7324
  dimension "d281" = 36.5762
  constraints: 4 end point, 3 point on line, 1 horizontal, 1 perpendicular
  measures "d279" distance between parallel lines of L2 L0
  measures "d280" distance of L0.start L0.end
  measures "d281" distance between parallel lines of L0 L4
sketch "Skizze48" plane through (-28.961, 0, -192.7131) normal (0, 0, 1) x (1, 0, 0)
  line L0 (0, 7) -> (0, 17) projected
  line L1 (70, 0) -> (70, 7) projected
  line L2 (0, 7) -> (70, 7)
  line L3 (70, 7) -> (70, 0)
  line L4 (70, 0) -> (0, 0)
  line L5 (0, 0) -> (0, 7)
  point P0 (28.961, 0)
  constraints: 8 end point, 2 parallel, 1 horizontal, 1 perpendicular
extrude "Extrusion40" add sketch "Skizze48" along normal blind 1.5
sketch "Skizze49" plane through (0, 17, 0) normal (0, 1, 0) x (1, 0, 0)
  point P0 (0, 0)
extrude "Extrusion41" add sketch "Skizze44" along normal blind 10 contours L13 L10 L11 L6
extrude "Extrusion42" add sketch "Skizze44" along normal blind 10 contours L15 L9 L1 L0 | L7 L21 L2 L1
